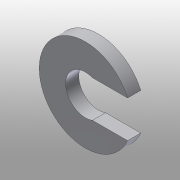
# Autodesk Inventor part: 500-168
Saved by Autodesk Inventor 2016 (Build 200138000, 138)
## iProperties
Created: 2015-04-18
Part Number: 500-168
Material: ABS Plastic
Document SubType Name: Modeling
Designer: Station9
Density: 1.06 g/cm^3
Appearance: Smooth - White
Mass: 0.0268667 g
Surface Area: 0.80955 cm^2
Volume: 0.0253459 cm^3
Author: Station9
Autodesk Inventor part; units mm, degrees
ref_plane "YZ Plane" through (0, 0, 0) normal (1, 0, 0) x (0, 1, 0)
ref_plane "XZ Plane" through (0, 0, 0) normal (0, 1, 0) x (-1, 0, 0)
ref_plane "XY Plane" through (0, 0, 0) normal (0, 0, 1) x (1, 0, 0)
sketch "Sketch1" plane through (0, 0, 0) normal (0, 1, 0) x (-1, 0, 0)
  line L0 (-0.5385, 1.4) -> (-3.2078, 1.4)
  line L1 (-7.0269, 1.4) -> (-7.0269, -1.4)
  line L2 (-3.2078, -1.4) -> (-0.5385, -1.4)
  line L3 (-0.5385, 1.4) -> (-7.0269, -1.4) construction
  line L4 (-7.0269, 1.4) -> (-0.5385, -1.4) construction
  arc A0 (-0.5385, -1.4) -> (-0.5385, 1.4) centre (0, 0) ccw
  arc A1 (-3.2078, -1.4) -> (-3.2078, 1.4) centre (0, 0) ccw
  point P0 (-3.7827, 0)
  dimension "d1" = 2.8
  dimension "d2" = 1.5
  constraints: 10 end point, 4 point on circle, 2 centre point, 2 coincident, 2 midpoint, 1 horizontal, 1 parallel, 1 perpendicular
  measures "d1" distance of L1.end L1.start
  measures "d2" radius of A0
extrude "Extrusion1" add sketch "Sketch1" along normal blind 3
sketch "Sketch2" plane through (0, 0, 0) normal (0, -1, 0) x (1, 0, 0)
  line L0 (0.5385, 1.4) -> (3.2078, 1.4) projected
  arc A0 (3.2078, 1.4) -> (3.2078, -1.4) centre (0, 0) ccw projected
  line L1 (3.2078, -1.4) -> (0.5385, -1.4) projected
  arc A1 (0.5385, 1.4) -> (0.5385, -1.4) centre (0, 0) ccw projected
extrude "Extrusion2" cut sketch "Sketch2" against normal blind 2
body "Solid1"
